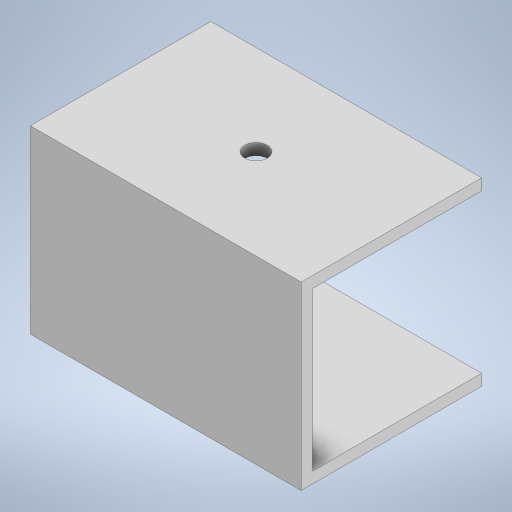
# Autodesk Inventor part: Gear Shell
Saved by Autodesk Inventor 2023 (Build 270158030, 158C)
## iProperties
Created: 2023-02-13
Part Number: Gear Shell
Material: Generic
Document SubType Name: Modeling
Designer: jeremyy
Density: 1 g/cm^3
Appearance: Default
Author: jeremyy
Autodesk Inventor part; units mm, degrees
ref_plane "YZ Plane" through (0, 0, 0) normal (1, 0, 0) x (0, 1, 0)
ref_plane "XZ Plane" through (0, 0, 0) normal (0, 1, 0) x (-1, 0, 0)
ref_plane "XY Plane" through (0, 0, 0) normal (0, 0, 1) x (1, 0, 0)
sketch "Sketch1" plane through (0, 0, 0) normal (0, 1, 0) x (-1, 0, 0)
  line L0 (0, 0) -> (76.2, 0)
  line L1 (76.2, 0) -> (76.2, -50.8)
  line L2 (76.2, -50.8) -> (0, -50.8)
  line L3 (0, -50.8) -> (0, 0)
  line L4 (76.2, -3.175) -> (0, -3.175)
  circle A0 centre (38.1, -25.4) radius 3.175
  dimension "d0" = 76.2
  dimension "d1" = 50.8
  dimension "d2" = 3.175
  dimension "d9" = 6.35
  dimension "d10" = 38.1
  dimension "d11" = 25.4
  constraints: 10 end point, 2 parallel, 2 perpendicular, 2 point on line, 1 centre point, 1 horizontal
  measures "d0" distance of L1.end L2.end
  measures "d1" distance of L0.end L1.end
  measures "d2" distance between parallel lines of L4 L0
  measures "d9" diameter of A0
  measures "d10" distance from line of L3 A0.centre
  measures "d11" distance from line of L2 A0.centre
extrude "Extrusion1" add sketch "Sketch1" along normal blind 3.175 contours L4 L1 L2 L3
extrude "Extrusion2" add sketch "Sketch1" along normal blind 50.8 contours L0 L1 L4 L3
sketch "Sketch2" plane through (0, 50.8, 0) normal (0, 1, 0) x (1, 0, 0)
  line L0 (0, 50.8) -> (-76.2, 50.8) projected
  line L1 (0, 0) -> (-76.2, 0)
  line L2 (-76.2, 0) -> (-76.2, 50.8)
  line L3 (-76.2, 50.8) -> (0, 50.8)
  line L4 (0, 50.8) -> (0, 0)
  line L5 (-76.2, 50.8) -> (-76.2, 3.175) projected
  line L6 (0, 3.175) -> (0, 50.8) projected
  line L7 (-76.2, 3.175) -> (0, 3.175)
  circle A0 centre (-38.1, 25.4) radius 3.175 projected
  circle A1 centre (-38.1, 25.4) radius 3.175
  dimension "d12" = 6.35
  constraints: 10 end point, 2 parallel, 2 perpendicular, 1 centre point, 1 coincident, 1 horizontal
  measures "d12" diameter of A1
extrude "Extrusion3" add sketch "Sketch2" against normal blind 3.175 contours L4 L7 L2 L0
body "Solid1"
